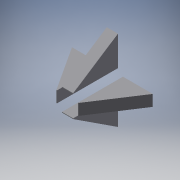
# Autodesk Inventor part: pilling
Saved by Autodesk Inventor 2016 (Build 200138000, 138)
## iProperties
Created: 2016-07-29
Part Number: pilling
Material: Generic
Document SubType Name: Modeling
Designer: Fred
Density: 1 g/cm^3
Appearance: Default
Author: Fred
Autodesk Inventor part; units mm, degrees
ref_plane "YZ Plane" through (0, 0, 0) normal (1, 0, 0) x (0, 1, 0)
ref_plane "XZ Plane" through (0, 0, 0) normal (0, 1, 0) x (-1, 0, 0)
ref_plane "XY Plane" through (0, 0, 0) normal (0, 0, 1) x (1, 0, 0)
sketch "Sketch1" plane through (0, 0, 0) normal (0, 0, 1) x (1, 0, 0)
  line L0 (40, 40) -> (40, -40) projected
  line L1 (-40, 40) -> (40, 40) projected
  line L2 (-40, -40) -> (-40, 40) projected
  line L3 (40, -40) -> (-40, -40) projected
  circle A0 centre (35, 35) radius 1.65 projected
  circle A1 centre (35, -35) radius 1.65 projected
  circle A2 centre (-35, -35) radius 1.65 projected
  circle A3 centre (-35, 35) radius 1.65 projected
  line L4 (0, -56) -> (0, 56)
  circle A4 centre (0, 0) radius 8 projected
  line L5 (-3.75, 27.0666) -> (3.75, 27.0666)
  line L6 (3.75, 27.0666) -> (3.75, 7.0666)
  line L7 (3.75, 7.0666) -> (-3.75, 7.0666)
  line L8 (-3.75, 7.0666) -> (-3.75, 27.0666)
  line L9 (-3.75, -7.0666) -> (3.75, -7.0666)
  line L10 (3.75, -7.0666) -> (3.75, -27.0666)
  line L11 (3.75, -27.0666) -> (-3.75, -27.0666)
  line L12 (-3.75, -27.0666) -> (-3.75, -7.0666)
  line L13 (-27.0666, 3.75) -> (-7.0666, 3.75)
  line L14 (-7.0666, 3.75) -> (-7.0666, -3.75)
  line L15 (-7.0666, -3.75) -> (-27.0666, -3.75)
  line L16 (-27.0666, -3.75) -> (-27.0666, 3.75)
  line L17 (7.0666, 3.75) -> (27.0666, 3.75)
  line L18 (27.0666, 3.75) -> (27.0666, -3.75)
  line L19 (27.0666, -3.75) -> (7.0666, -3.75)
  line L20 (7.0666, -3.75) -> (7.0666, 3.75)
  line L21 (-56, 0) -> (56, 0)
  point P0 (0, 0)
  dimension "d0" = 20
  dimension "d1" = 7.5
  dimension "d2" = 3.75
  dimension "d3" = 20
  dimension "d4" = 7.5
  dimension "d9" = 3.75
  dimension "d10" = 7.5
  dimension "d11" = 20
  dimension "d12" = 20
  dimension "d13" = 7.5
  dimension "d14" = 3.75
  constraints: 36 end point, 8 parallel, 5 horizontal, 4 perpendicular, 4 point on circle, 1 point on line, 1 vertical, 4 other
  measures "d0" distance of L5.end L6.end
  measures "d1" distance of L5.start L5.end
  measures "d2" distance between parallel lines of L6 L4
  measures "d3" distance of L9.end L10.end
  measures "d4" distance of L9.start L9.end
  measures "d9" distance between parallel lines of L4 L10
  measures "d10" distance of L15.end L13.start
  measures "d11" distance of L13.start L13.end
  measures "d12" distance of L17.start L17.end
  measures "d13" distance of L17.end L18.end
  measures "d14" distance between parallel lines of L19 L21
extrude "Extrusion1" add sketch "Sketch1" along normal blind 30 contours L21 A4 L17 L18 | L18 L19 A4 L21 | L5 L6 A4 L4 | L4 A4 L8 L5 | L21 L20 A4 | A4 L20 L21 | A4 L7 L4 | L4 L7 A4 | L11 L12 A4 L4 | L4 A4 L10 L11 | L21 A4 L15 L16 | L16 L13 A4 L21 | A4 L9 L4 | L4 L9 A4 | L21 L14 A4 | A4 L14 L21
chamfer "Chamfer1" distance 19.5555 angle 56.9 1 edges at (0, 27.0666, 30) measured on face at (-1.25, 20.4, 30)
chamfer "Chamfer2" distance 19.5555 angle 56.9 1 edges at (27.0666, 0, 30) measured on face at (13.7333, 1.25, 30)
chamfer "Chamfer3" distance 19.5555 angle 56.9 1 edges at (-27.0666, 0, 30) measured on face at (-20.4, 1.25, 30)
chamfer "Chamfer4" distance 19.5555 angle 56.9 1 edges at (0, -27.0666, 30) measured on face at (-1.25, -13.7333, 30)
equation "\"d2\" = 0.5 * d1"
equation "\"d3\" = d0"
equation "\"d4\" = d1"
equation "\"d9\" = d2"
equation "\"d10\" = d1"
equation "\"d11\" = d0"
equation "\"d12\" = d0"
equation "\"d13\" = d1"
equation "\"d14\" = d2"
body "Solid1"
